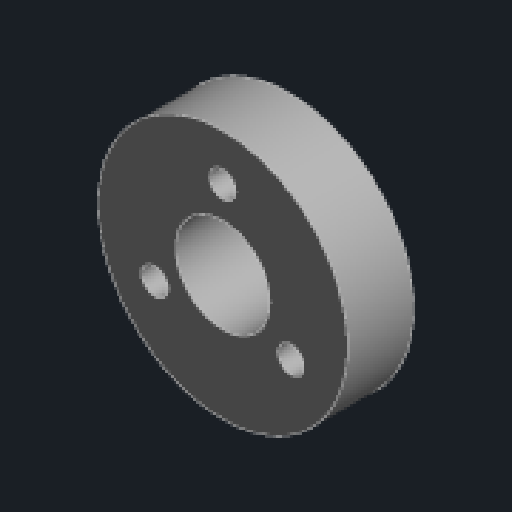
# Autodesk Inventor part: LegMotorSpacer
Saved by Autodesk Inventor 2025.2 (Build 292293000, 293)
## iProperties
Created: 2025-10-11
Part Number: LegMotorSpacer
Material: Generic
Document SubType Name: Modeling
Designer: valer
Density: 1 g/cm^3
Appearance: Default
Author: valer
Autodesk Inventor part; units mm, degrees
ref_plane "YZ Plane" through (0, 0, 0) normal (1, 0, 0) x (0, 1, 0)
ref_plane "XZ Plane" through (0, 0, 0) normal (0, 1, 0) x (-1, 0, 0)
sketch "Sketch1" plane through (0, 0, 0) normal (0, 0, 1) x (1, 0, 0)
  circle A0 centre (0, 20.7846) radius 3.5 projected
  circle A1 centre (-18, -10.3923) radius 3.5 projected
  circle A2 centre (18, -10.3923) radius 3.5 projected
  circle A3 centre (0, 0) radius 6.75 construction
  circle A4 centre (0, 0) radius 12.5
  circle A5 centre (0, 0) radius 33 projected
  point P0 (0, 0)
  dimension "d0" = 25
  constraints: 1 centre point, 1 coincident
  measures "d0" diameter of A4
ref_plane "Work Plane1" through (-191.7635, -303.2503, 17.5) normal (0, 0, -1) x (-0.1566, 0.9877, 0)
extrude "Extrusion1" add sketch "Sketch1" along normal up to surface (17.5 mm away)
body "Solid1"
